PCB Lock (Autodesk Fusion 360 design; units mm, degrees)
Autodesk Fusion 360 part; units mm, degrees
sketch "Sketch1" plane through (0, 0, 0) normal (0, 0, 1) x (1, 0, 0)
  circle A0 centre (0, 0) radius 8.175
  circle A1 centre (0, 0) radius 6.5
  dimension "d1" = 16.35
  dimension "d2" = 13
  constraint coincident A0.centre A1.centre
  constraint concentric A0 A1
  measures "d1" diameter of A0
  measures "d2" diameter of A1
extrude "Extrude1" add sketch "Sketch1" along normal blind 1.5
sketch "Sketch2" plane through (0, 0, 1.5) normal (0, 0, 1) x (-1, 0, 0)
  circle A0 centre (0, 0) radius 6.5
  circle A1 centre (0, 0) radius 8.175
  line L0 (4, 0) -> (-4, 0)
  line L1 (-4, 0) -> (-4, 8.5)
  line L2 (-4, 8.5) -> (4, 8.5)
  line L3 (4, 8.5) -> (4, 0)
  dimension "d5" = 8
  dimension "d6" = 4
  dimension "d7" = 8.5
  constraint horizontal L0
  constraint vertical L1
  constraint horizontal L2
  constraint vertical L3
  constraint horizontal A0.centre L0.end
  measures "d5" distance of L1 L3
  measures "d6" distance of A0.centre L1
  measures "d7" distance of L0 L2
extrude "Extrude2" cut sketch "Sketch2" against normal blind 2 contours A0 A1 L1 L3 picked at (3.0865, 6.9432)
fillet "Fillet1" radius 2.5 2 edges at (-4, -5.1235, 0.75) (4, -5.1235, 0.75)
sketch "Sketch3" plane through (0, 0, 1.5) normal (0, 0, 1) x (-1, 0, 0)
  arc A0 (-4.6944, 4.4958) -> (-4, 6.2249) centre (-6.5, 6.2249) ccw
  line L0 (-4, 6.2249) -> (-4, 7.1296)
  arc A1 (-4, 7.1296) -> (4, 7.1296) centre (0, 0) ccw
  line L1 (4, 7.1296) -> (4, 6.2249)
  arc A2 (4, 6.2249) -> (4.6944, 4.4958) centre (6.5, 6.2249) ccw
  arc A3 (-4.6944, 4.4958) -> (4.6944, 4.4958) centre (0, 0) ccw
  line L2 (10.6029, -1) -> (-9.8214, -1)
  line L3 (-9.8214, -1) -> (-9.8214, 1)
  line L4 (-9.8214, 1) -> (10.6029, 1)
  line L5 (10.6029, 1) -> (10.6029, -1)
  circle A4 centre (0, 0) radius 8.675
  dimension "d12" = 2
  dimension "d13" = 1
  dimension "d14" = 17.35
  constraint horizontal L2
  constraint vertical L3
  constraint horizontal L4
  constraint vertical L5
  constraint coincident A1.centre A3.centre
  measures "d12" distance of L2 L4
  measures "d13" distance of A1.centre L4
  measures "d14" diameter of A4
extrude "Extrude3" add sketch "Sketch3" against normal blind 1.5 contours A1 L2 L4 A4 | A1 L2 L4 A4
extrude "Extrude4" cut 1 faces at (7.4278, 1.6054, 1.5) along direction (0, 0, -1) blind 0.15
